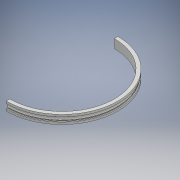
# Autodesk Inventor part: 母摩-半圓
Saved by Autodesk Inventor 2018 (Build 220112000, 112)
## iProperties
Created: 2026-01-23
Part Number: 母摩-半圓
Material: 一般
Document SubType Name: Modeling
Designer: User
Density: 1 g/cm^3
Appearance: 預設
Mass: 769.932 g
Surface Area: 1487.57 cm^2
Volume: 769.932 cm^3
Author: User
Autodesk Inventor part; units mm, degrees
ref_plane "YZ Plane" through (0, 0, 0) normal (1, 0, 0) x (0, 1, 0)
ref_plane "XZ Plane" through (0, 0, 0) normal (0, 1, 0) x (-1, 0, 0)
ref_plane "XY Plane" through (0, 0, 0) normal (0, 0, 1) x (1, 0, 0)
sketch "草圖1" plane through (0, 0, 0) normal (1, 0, 0) x (0, 1, 0)
  line L0 (-297, 25) -> (-317, 25)
  line L1 (-317, 25) -> (-317, -25)
  line L2 (-317, -25) -> (-297, -25)
  line L3 (-297, -25) -> (-297, 25)
  line L4 (-312, 12.85) -> (-317, 12.85)
  line L5 (-317, -12.85) -> (-312, -12.85)
  line L6 (-307.8, -12.85) -> (-307.8, 12.85) construction
  arc A0 (-310.3, -7.8899) -> (-310.3, 7.8899) centre (-321.5, 0) ccw
  line L7 (-310.3, 11.15) -> (-310.3, 7.8899)
  line L8 (-310.3, -7.8899) -> (-310.3, -11.15)
  arc A1 (-310.1299, -7.6427) -> (-310.3, -8.2006) centre (-309.3, -8.2006) ccw
  arc A2 (-310.3, 8.2006) -> (-310.1299, 7.6427) centre (-309.3, 8.2006) ccw
  arc A3 (-310.3, 11.15) -> (-312, 12.85) centre (-312, 11.15) ccw
  arc A4 (-312, -12.85) -> (-310.3, -11.15) centre (-312, -11.15) ccw
  line L9 (0, 0) -> (0, 24.4036)
  dimension "d0" = 317
  dimension "d1" = 25
  dimension "d3" = 50
  dimension "d4" = 20
  dimension "d5" = 9.2
  dimension "d6" = 12.85
  dimension "d7" = 25.7
  dimension "d8" = 27.4
  dimension "d9" = 0
  dimension "d10" = 2.5
  dimension "d11" = 2.5
  dimension "d12" = 2
  dimension "d13" = 2
  dimension "d14" = 3.4
  dimension "d15" = 3.4
  constraints: 20 end point, 12 point on circle, 9 tangent, 5 centre point, 4 point on line, 3 parallel, 3 vertical, 2 horizontal, 1 perpendicular
  measures "d0" distance from line of L9.start L1
  measures "d1" distance from line of L9.start L2
  measures "d3" distance between parallel lines of L2 L0
  measures "d4" distance between parallel lines of L1 L3
  measures "d5" distance between parallel lines of L1 L6
  measures "d6" distance from line of L9.start L4
  measures "d7" distance between parallel lines of L4 L5
  measures "d8" diameter of A0
  measures "d9" vertical distance of L9.start A0.centre
  measures "d10" distance between parallel lines of L6 L7
  measures "d11" distance between parallel lines of L6 L8
  measures "d12" diameter of A2
  measures "d13" diameter of A1
  measures "d14" diameter of A3
  measures "d15" diameter of A4
revolve "迴轉1" add sketch "草圖1" angle 180 about axis through (0, 0, 0) along (0, 0, 1) contours L3 L2 L1 L5 A4 L8 A1 A0 A2 L7 A3 L4 L0
